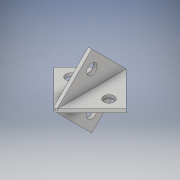
# Autodesk Inventor part: MainStructure
Saved by Autodesk Inventor 2018.3 (Build 223284000, 284)
## iProperties
Created: 2020-03-24
Part Number: MainStructure
Material: Generic
Document SubType Name: Modeling
Designer: ToreDenStore
Density: 1 g/cm^3
Appearance: Default
Author: ToreDenStore
Autodesk Inventor part; units mm, degrees
ref_plane "YZ Plane" through (0, 0, 0) normal (1, 0, 0) x (0, 1, 0)
ref_plane "XZ Plane" through (0, 0, 0) normal (0, 1, 0) x (-1, 0, 0)
ref_plane "XY Plane" through (0, 0, 0) normal (0, 0, 1) x (1, 0, 0)
sketch "Sketch1" plane through (0, 0, 0) normal (0, 1, 0) x (-1, 0, 0)
  point P0 (0, 0)
sketch "Sketch2" plane through (0, 0, 0) normal (0, 1, 0) x (-1, 0, 0)
  line L0 (0, 0) -> (0, -100)
  line L1 (0, -100) -> (100, 0)
  line L2 (100, 0) -> (0, 0) construction
  line L3 (0, 0) -> (0, 100)
  line L4 (0, 100) -> (100, 0)
  circle A0 centre (50, 0) radius 15
  dimension "d0" = 100
  dimension "d1" = 45
  dimension "d2" = 30
  dimension "d3" = 50
  constraints: 10 end point, 1 centre point, 1 midpoint, 1 perpendicular, 1 symmetric about line, 1 vertical
  measures "d0" distance of L0.start L0.end
  measures "d1" angle of L0 L1
  measures "d2" diameter of A0
  measures "d3" distance from line of L3 A0.centre
extrude "Extrusion1" add sketch "Sketch2" along normal blind 10
sketch "Sketch3" plane through (0, 0, 100) normal (1, 0, 0) x (0, 0, -1)
  line L0 (0, 0) -> (200, 0) projected
  line L1 (200, 0) -> (200, 10) projected
  line L2 (0, 10) -> (200, 10) projected
  line L3 (0, 0) -> (0, 10) projected
  point P0 (100, 0)
extrude "Extrusion2" add sketch "Sketch3" along normal blind 10
sketch "Sketch4" plane through (0, 0, 100) normal (0, 0, 1) x (1, 0, 0)
  circle A0 centre (5, 5) radius 2
  line L0 (0, 10) -> (10, 10) projected
  line L1 (10, 10) -> (10, 0) projected
  point P0 (0, 0)
  dimension "d8" = 4
  dimension "d9" = 5
  dimension "d10" = 5
  constraints: 1 centre point
  measures "d8" diameter of A0
  measures "d9" distance from line of A0.centre L0
  measures "d10" distance from line of A0.centre L1
extrude "Extrusion3" cut sketch "Sketch4" against normal blind 252.8875
pattern_circular "Circular Pattern1" count 4 over 360 about axis through (5, 5, 100) along (0, 0, -1) of "Extrusion1"
body "Solid1"
